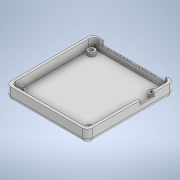
# Autodesk Inventor part: Enclosure Box
Saved by Autodesk Inventor 2021 (Build 250183000, 183)
## iProperties
Created: 2021-06-04
Part Number: Enclosure Box
Material: Generic
Document SubType Name: Modeling
Designer: Anton
Density: 1 g/cm^3
Appearance: Default
Author: Anton
Autodesk Inventor part; units mm, degrees
ref_plane "YZ Plane" through (0, 0, 0) normal (1, 0, 0) x (0, 1, 0)
ref_plane "XZ Plane" through (0, 0, 0) normal (0, 1, 0) x (-1, 0, 0)
ref_plane "XY Plane" through (0, 0, 0) normal (0, 0, 1) x (1, 0, 0)
sketch "Sketch2" plane through (0, 0, 0) normal (0, 1, 0) x (-1, 0, 0)
  line L0 (0, 0) -> (62, 0)
  line L1 (62, 0) -> (62, -66)
  line L2 (62, -66) -> (0, -66)
  line L3 (0, -66) -> (0, 0)
  circle A0 centre (58.15, -9.3) radius 1.5
  circle A1 centre (57.35, -60.86) radius 1.5
  circle A2 centre (3, -4.5) radius 1.5
  circle A3 centre (3, -61.9) radius 1.5
  circle A4 centre (3, -4.5) radius 3
  circle A5 centre (58.15, -9.3) radius 3
  circle A6 centre (57.35, -60.86) radius 3
  circle A7 centre (3, -61.9) radius 3
  line L4 (63, 20) -> (-1, 20)
  line L5 (-1, 20) -> (-1, -86)
  line L6 (-1, -86) -> (63, -86)
  line L7 (63, -86) -> (63, 20)
  dimension "d14" = 66
  dimension "d15" = 62
  dimension "d16" = 3
  dimension "d17" = 3
  dimension "d18" = 3
  dimension "d19" = 3
  dimension "d20" = 3
  dimension "d21" = 4.5
  dimension "d22" = 6
  dimension "d23" = 3
  dimension "d24" = 57.4
  dimension "d25" = 54.35
  dimension "d26" = 0.8
  dimension "d27" = 51.56
  dimension "d28" = 4.8
  dimension "d29" = 6
  dimension "d30" = 6
  dimension "d31" = 6
  dimension "d32" = 20
  dimension "d33" = 20
  dimension "d34" = 1
  dimension "d35" = 1
  constraints: 16 end point, 8 centre point, 4 coincident, 4 parallel, 2 horizontal, 2 perpendicular
  measures "d14" distance between parallel lines of L2 L0
  measures "d15" distance between parallel lines of L3 L1
  measures "d16" diameter of A0
  measures "d17" diameter of A1
  measures "d18" diameter of A3
  measures "d19" diameter of A2
  measures "d20" distance from line of L3 A2.centre
  measures "d21" distance from line of A2.centre L0
  measures "d22" diameter of A4
  measures "d23" distance from line of L3 A3.centre
  measures "d24" distance of A2.centre A3.centre
  measures "d25" horizontal distance of A1.centre A3.centre
  measures "d26" horizontal distance of A1.centre A0.centre
  measures "d27" vertical distance of A1.centre A0.centre
  measures "d28" vertical distance of A2.centre A0.centre
  measures "d29" diameter of A5
  measures "d30" diameter of A6
  measures "d31" diameter of A7
  measures "d32" distance between parallel lines of L4 L0
  measures "d33" distance between parallel lines of L2 L6
  measures "d34" distance between parallel lines of L7 L1
  measures "d35" distance between parallel lines of L3 L5
extrude "Extrusion1" add sketch "Sketch2" along normal blind 2 contours A4 | A7 | L0 L1 L2 L3 | A0 | A1 | A2 | A3 | A5 | A6
sketch "Sketch4" plane through (0, 2, 0) normal (0, 1, 0) x (1, 0, 0)
  line L0 (-62, 66) -> (0, 66)
  line L1 (0, 66) -> (0, 0)
  line L2 (0, 0) -> (-62, 0)
  line L3 (-62, 0) -> (-62, 66)
  circle A0 centre (-3.85, 56.7) radius 1.5
  circle A1 centre (-4.65, 5.14) radius 1.5
  circle A2 centre (-59, 61.5) radius 1.5
  circle A3 centre (-59, 4.1) radius 1.5
  circle A4 centre (-59, 61.5) radius 3
  circle A5 centre (-3.85, 56.7) radius 3
  circle A6 centre (-4.65, 5.14) radius 3
  circle A7 centre (-59, 4.1) radius 3
  point P0 (0, 0)
  dimension "d38" = 66
  dimension "d40" = 3
  dimension "d41" = 3
  dimension "d42" = 3
  dimension "d43" = 3
  dimension "d44" = 3
  dimension "d45" = 4.5
  dimension "d46" = 6
  dimension "d47" = 3
  dimension "d48" = 57.4
  dimension "d50" = 0.8
  dimension "d51" = 51.56
  dimension "d52" = 4.8
  dimension "d53" = 6
  dimension "d54" = 6
  dimension "d55" = 6
  constraints: 8 centre point, 8 end point, 4 coincident, 2 parallel, 1 horizontal, 1 perpendicular
  measures "d38" distance between parallel lines of L2 L0
  measures "d40" diameter of A0
  measures "d41" diameter of A1
  measures "d42" diameter of A3
  measures "d43" diameter of A2
  measures "d44" distance from line of L3 A2.centre
  measures "d45" distance from line of A2.centre L0
  measures "d46" diameter of A4
  measures "d47" distance from line of L3 A3.centre
  measures "d48" distance of A2.centre A3.centre
  measures "d50" horizontal distance of A1.centre A0.centre
  measures "d51" vertical distance of A1.centre A0.centre
  measures "d52" vertical distance of A2.centre A0.centre
  measures "d53" diameter of A5
  measures "d54" diameter of A6
  measures "d55" diameter of A7
extrude "Extrusion2" add sketch "Sketch4" along normal blind 3 contours A4 | A7 | A0 | A1 | A2 | A3 | A5 | A6
sketch "Sketch69" plane through (-59, 5, -4.1) normal (0, 1, 0) x (1, 0, 0)
  circle A0 centre (54.35, 1.04) radius 3 projected
  circle A1 centre (54.35, 1.04) radius 1.25
  circle A2 centre (55.15, 52.6) radius 3 projected
  circle A3 centre (55.15, 52.6) radius 1.25
  circle A4 centre (0, 57.4) radius 3 projected
  circle A5 centre (0, 57.4) radius 1.25
  circle A6 centre (0, 0) radius 3 projected
  circle A7 centre (0, 0) radius 1.25
  point P0 (59, -4.1)
  point P1 (-3, 57.4)
  point P2 (-3, 0)
  dimension "d432" = 2.5
  dimension "d433" = 2.5
  dimension "d434" = 2.5
  dimension "d435" = 2.5
  constraints: 4 centre point, 4 coincident, 2 horizontal alignment
  measures "d432" diameter of A7
  measures "d433" diameter of A5
  measures "d434" diameter of A3
  measures "d435" diameter of A1
extrude "Extrusion56" add sketch "Sketch69" along normal blind 3 contours A1 | A3 | A5 | A7
sketch "Sketch72" plane through (0, 2, 0) normal (0, 1, 0) x (1, 0, 0)
  line L0 (-62, 66) -> (-62, 0) projected
  line L1 (-62, 66) -> (-65, 66)
  line L2 (-65, 66) -> (-65, 0)
  line L3 (-65, 0) -> (-62, 0)
  line L4 (-62, 0) -> (-62, 66)
  circle A0 centre (-59, 61.5) radius 1.25 projected
  line L5 (0, 66) -> (-62, 66) projected
  line L6 (-62, 0) -> (0, 0) projected
  line L7 (0, 0) -> (2.15, 0)
  line L8 (2.15, 0) -> (2.15, 66)
  line L9 (2.15, 66) -> (0, 66)
  line L10 (0, 66) -> (0, 0)
  circle A1 centre (-3.85, 56.7) radius 1.25 projected
  line L11 (-65, 66) -> (2.15, 66)
  line L12 (2.15, 66) -> (2.15, 68.5)
  line L13 (2.15, 68.5) -> (-65, 68.5)
  line L14 (-65, 68.5) -> (-65, 66)
  line L15 (-65, 0) -> (2.15, 0)
  line L16 (2.15, 0) -> (2.15, -3)
  line L17 (2.15, -3) -> (-65, -3)
  line L18 (-65, -3) -> (-65, 0)
  circle A2 centre (-59, 4.1) radius 1.25 projected
  dimension "d446" = 6
  dimension "d447" = 0
  dimension "d448" = 6
  dimension "d449" = 7
  dimension "d450" = 7.1
  dimension "d464" = 0
  dimension "d465" = 0
  constraints: 32 end point, 8 parallel, 4 horizontal, 4 perpendicular, 1 point on line
  measures "d446" distance from line of A0.centre L2
  measures "d447" distance between parallel lines of L5 L1
  measures "d448" distance from line of L8 A1.centre
  measures "d449" distance from line of A0.centre L13
  measures "d450" distance from line of L17 A2.centre
  measures "d464" distance between parallel lines of L8 L12
  measures "d465" distance between parallel lines of L8 L16
extrude "Extrusion58" add sketch "Sketch72" against normal blind 2 contours L0 L3 L2 L1 | L1 L14 L13 L12 L9 L5 | L6 L7 L16 L17 L18 L3 | L9 L8 L7 L10
sketch "Sketch73" plane through (0, 2, 0) normal (0, 1, 0) x (1, 0, 0)
  line L0 (2.15, -3) -> (-65, -3) projected
  line L1 (-65, 68.5) -> (2.15, 68.5) projected
  line L2 (-65, -3) -> (2.15, -3)
  line L3 (2.15, -3) -> (2.15, 68.5)
  line L4 (2.15, 68.5) -> (-65, 68.5)
  line L5 (-65, 68.5) -> (-65, -3)
  line L6 (-63, -1) -> (0.15, -1)
  line L7 (0.15, -1) -> (0.15, 66.5)
  line L8 (0.15, 66.5) -> (-63, 66.5)
  line L9 (-63, 66.5) -> (-63, -1)
  point P0 (0, 0)
  point P1 (2.15, -3)
  dimension "d453" = 2
  constraints: 16 end point, 4 parallel, 2 perpendicular, 1 horizontal, 3 other
  measures "d453" distance between parallel lines of L5 L9
extrude "Extrusion59" add sketch "Sketch73" along normal blind 6
sketch "Sketch74" plane through (0, 8, 0) normal (0, 1, 0) x (1, 0, 0)
  line L0 (6.1553, 52.4) -> (-1.961, 52.4)
  line L1 (-1.961, 52.4) -> (-1.961, 40.4)
  line L2 (-1.961, 40.4) -> (6.1553, 40.4)
  line L3 (6.1553, 40.4) -> (6.1553, 52.4)
  line L4 (-3.5, 77.4858) -> (-56, 77.4858)
  line L5 (-56, 77.4858) -> (-56, 63.7045)
  line L6 (-56, 63.7045) -> (-3.5, 63.7045)
  line L7 (-3.5, 63.7045) -> (-3.5, 77.4858)
  circle A0 centre (-59, 61.5) radius 1.25 projected
  line L8 (0.15, -1) -> (0.15, 66.5) projected
  line L9 (-63, 67.5) -> (0.15, 67.5)
  line L10 (0.15, 67.5) -> (0.15, 64.6943)
  line L11 (0.15, 64.6943) -> (-63, 64.6943)
  line L12 (-63, 64.6943) -> (-63, 67.5)
  line L13 (-63, 66.5) -> (0.15, 66.5) projected
  circle A1 centre (-3.85, 56.7) radius 1.25 projected
  point P0 (0, 0)
  point P1 (-56, 64.6943)
  point P2 (-3.5, 64.6943)
  point P3 (-56, 66.5)
  point P4 (-56, 67.5)
  point P5 (-3.5, 66.5)
  point P6 (0.15, 66.5)
  point P7 (-3.5, 67.5)
  dimension "d457" = 52.5
  dimension "d458" = 1
  dimension "d459" = 4.3
  dimension "d460" = 12
  dimension "d463" = 3
  constraints: 24 end point, 6 parallel, 3 horizontal, 3 perpendicular, 1 point on line
  measures "d457" distance between parallel lines of L7 L5
  measures "d458" distance between parallel lines of L13 L9
  measures "d459" distance from line of L0 A1.centre
  measures "d460" distance between parallel lines of L0 L2
  measures "d463" distance from line of L5 A0.centre
extrude "Extrusion60" cut sketch "Sketch74" against normal blind 3 contours L3 L2 L8 L0 | L8 L2 L1 L0 | L13 L7 L9 L10 | L11 L5 L13 L7 | L13 L5 L9 L7 | L9 L5 L4 L7 | L13 L12 L9 L5
sketch "Sketch75" plane through (0, 5, 0) normal (0, 1, 0) x (1, 0, 0)
  line L0 (-56, 68.5) -> (-3.5, 68.5) projected
  line L1 (-56, 68.5) -> (-3.5, 68.5)
  line L2 (-3.5, 68.5) -> (-3.5, 67.5)
  line L3 (-3.5, 67.5) -> (-56, 67.5)
  line L4 (-56, 67.5) -> (-56, 68.5)
  point P0 (0, 0)
  point P1 (-3.5, 68.5)
  constraints: 8 end point, 2 parallel, 1 horizontal, 1 perpendicular
extrude "Extrusion61" add sketch "Sketch75" along normal blind 1.5
sketch "Sketch77" plane through (0, 5, 0) normal (0, 1, 0) x (1, 0, 0)
  line L0 (2.15, 52.4) -> (2.15, 68.5) projected
  line L1 (2.15, 40.4) -> (0.15, 40.4) projected
  line L2 (2.15, 52.4) -> (1.15, 52.4)
  line L3 (1.15, 52.4) -> (1.15, 40.4)
  line L4 (1.15, 40.4) -> (2.15, 40.4)
  line L5 (2.15, 40.4) -> (2.15, 52.4)
  point P0 (0, 0)
  dimension "d469" = 1
  constraints: 8 end point, 2 parallel, 1 horizontal, 1 midpoint, 1 perpendicular
  measures "d469" distance between parallel lines of L5 L3
extrude "Extrusion62" add sketch "Sketch77" along normal blind 1.5
sketch "Sketch78" plane through (0, 8, 0) normal (0, 1, 0) x (1, 0, 0)
  line L0 (2.15, 40.4) -> (0.15, 40.4) projected
  line L1 (0.15, 40.4) -> (0.15, -1) projected
  line L2 (0.15, -1) -> (-63, -1) projected
  line L3 (-63, -1) -> (-63, 67.5) projected
  line L4 (-63, 67.5) -> (-56, 67.5) projected
  line L5 (-56, 67.5) -> (-56, 68.5) projected
  line L6 (-56, 68.5) -> (-65, 68.5) projected
  line L7 (-65, 68.5) -> (-65, -3) projected
  line L8 (-65, -3) -> (2.15, -3) projected
  line L9 (2.15, -3) -> (2.15, 40.4) projected
  line L10 (0.15, 52.4) -> (2.15, 52.4) projected
  line L11 (2.15, 52.4) -> (2.15, 68.5) projected
  line L12 (2.15, 68.5) -> (-3.5, 68.5) projected
  line L13 (-3.5, 68.5) -> (-3.5, 67.5) projected
  line L14 (-3.5, 67.5) -> (0.15, 67.5) projected
  line L15 (0.15, 67.5) -> (0.15, 52.4) projected
  point P0 (0, 0)
extrude "Extrusion63" add sketch "Sketch78" along normal blind 2
sketch "Sketch80" plane through (0, 10, 0) normal (0, 1, 0) x (1, 0, 0)
  line L0 (2.15, -3) -> (-65, -3) projected
  line L1 (-1.85, -3) -> (-61, -3)
  line L2 (-65, 1) -> (-65, 64.5)
  line L3 (-61, 68.5) -> (-1.85, 68.5)
  line L4 (2.15, 64.5) -> (2.15, 1)
  line L5 (-68.7627, 72.319) -> (6.3795, 72.319)
  line L6 (6.3795, 72.319) -> (6.3795, -5.0493)
  line L7 (6.3795, -5.0493) -> (-68.7627, -5.0493)
  line L8 (-68.7627, -5.0493) -> (-68.7627, 72.319)
  arc A0 (-61, 68.5) -> (-65, 64.5) centre (-61, 64.5) ccw
  arc A1 (2.15, 64.5) -> (-1.85, 68.5) centre (-1.85, 64.5) ccw
  arc A2 (-1.85, -3) -> (2.15, 1) centre (-1.85, 1) ccw
  arc A3 (-65, 1) -> (-61, -3) centre (-61, 1) ccw
  point P0 (0, 0)
  point P1 (-65, 68.5)
  dimension "d475" = 4
  constraints: 16 end point, 8 point on circle, 8 tangent, 4 centre point, 4 parallel, 4 point on line, 3 equal radius, 2 horizontal, 2 perpendicular
  measures "d475" radius of A0
extrude "Extrusion64" cut sketch "Sketch80" against normal blind 10
sketch "Sketch81" plane through (0, 10, 0) normal (0, 1, 0) x (1, 0, 0)
  line L0 (0.15, 40.4) -> (0.15, -1) projected
  line L1 (-63, 66.5) -> (-63, 67.5) projected
  line L2 (-3.85, -1) -> (-59, -1)
  line L3 (-63, 3) -> (-63, 63.5)
  line L4 (-59, 67.5) -> (-3.85, 67.5)
  line L5 (0.15, 63.5) -> (0.15, 3)
  arc A0 (-59, 67.5) -> (-63, 63.5) centre (-59, 63.5) ccw
  arc A1 (0.15, 63.5) -> (-3.85, 67.5) centre (-3.85, 63.5) ccw
  arc A2 (-3.85, -1) -> (0.15, 3) centre (-3.85, 3) ccw
  arc A3 (-63, 3) -> (-59, -1) centre (-59, 3) ccw
  line L6 (0.15, -1) -> (-63, -1) projected
  line L7 (-63, 67.5) -> (0.15, 67.5)
  line L8 (0.15, 67.5) -> (0.15, -1)
  line L9 (0.15, -1) -> (-63, -1)
  line L10 (-63, -1) -> (-63, 67.5)
  point P0 (0, 0)
  dimension "d478" = 4
  constraints: 16 end point, 8 point on circle, 8 tangent, 4 centre point, 4 parallel, 4 point on line, 3 equal radius, 2 horizontal, 2 perpendicular
  measures "d478" radius of A0
extrude "Extrusion65" add sketch "Sketch81" against normal up to surface (8 mm away) contours L0 L6 A2 | A1 L7 L8 | L6 L10 A3 | A0 L10 L1 L7
sketch "Sketch82" plane through (0, 0, 0) normal (0, -1, 0) x (1, 0, 0)
  arc A0 (-61, 3) -> (-65, -1) centre (-61, -1) ccw projected
  line L0 (-65, -1) -> (-65, -64.5) projected
  arc A1 (-65, -64.5) -> (-61, -68.5) centre (-61, -64.5) ccw projected
  line L1 (-61, -68.5) -> (-1.85, -68.5) projected
  arc A2 (-1.85, -68.5) -> (2.15, -64.5) centre (-1.85, -64.5) ccw projected
  line L2 (2.15, -64.5) -> (2.15, -1) projected
  arc A3 (2.15, -1) -> (-1.85, 3) centre (-1.85, -1) ccw projected
  line L3 (-1.85, 3) -> (-61, 3) projected
  point P0 (0, 0)
extrude "Extrusion66" add sketch "Sketch82" along normal blind 1
sketch "Sketch83" plane through (-59, 5, -4.1) normal (0, 1, 0) x (1, 0, 0)
  circle A0 centre (54.35, 1.04) radius 1.25 projected
  circle A1 centre (54.35, 1.04) radius 1.5
  circle A2 centre (55.15, 52.6) radius 1.25 projected
  circle A3 centre (55.15, 52.6) radius 1.5
  circle A4 centre (0, 57.4) radius 1.25 projected
  circle A5 centre (0, 57.4) radius 1.5
  circle A6 centre (0, 0) radius 1.25 projected
  circle A7 centre (0, 0) radius 1.5
  point P0 (59, -4.1)
  dimension "d484" = 3
  dimension "d486" = 3
  dimension "d487" = 3
  dimension "d488" = 3
  constraints: 4 centre point, 4 coincident
  measures "d484" diameter of A7
  measures "d486" diameter of A5
  measures "d487" diameter of A3
  measures "d488" diameter of A1
extrude "Extrusion67" cut sketch "Sketch83" along normal mid plane 1011 contours A0 | A1 | A2 | A3 | A4 | A5 | A6 | A7
fillet "Fillet13" radius 4 8 edges at (0.9784, -1, -67.3284) (2.15, -1, -32.75) (0.9784, -1, 1.8284) (-31.425, -1, 3) (-63.8284, -1, 1.8284) (-65, -1, -32.75) (-63.8284, -1, -67.3284) (-31.425, -1, -68.5)
sketch "Sketch84" plane through (0, -1, 0) normal (0, -1, 0) x (1, 0, 0)
  circle A0 centre (-4.65, -5.14) radius 3 projected
  circle A1 centre (-4.65, -5.14) radius 3
  circle A2 centre (-3.85, -56.7) radius 1.5 projected
  circle A3 centre (-3.85, -56.7) radius 3
  circle A4 centre (-59, -61.5) radius 1.5 projected
  circle A5 centre (-59, -61.5) radius 3
  circle A6 centre (-59, -4.1) radius 1.5 projected
  circle A7 centre (-59, -4.1) radius 3
  point P0 (0, 0)
  dimension "d492" = 6
  dimension "d493" = 6
  dimension "d494" = 6
  dimension "d495" = 6
  constraints: 4 centre point, 4 coincident
  measures "d492" diameter of A7
  measures "d493" diameter of A5
  measures "d494" diameter of A3
  measures "d495" diameter of A1
extrude "Extrusion68" cut sketch "Sketch84" against normal blind 2.5 contours A0 | A2 | A3 | A4 | A5 | A7
sketch "Sketch86" plane through (-3.5, 6.5, -68.5) normal (0, 0, -1) x (-1, 0, 0)
  line L0 (0, 0) -> (0, 3.5) projected
  line L1 (57.5, -3.5) -> (-1.65, -3.5) projected
  line L2 (0, 0) -> (52.5, 0)
  line L3 (52.5, 0) -> (52.5, -3.5)
  line L4 (52.5, -3.5) -> (0, -3.5)
  line L5 (0, -3.5) -> (0, 0)
  line L6 (52.5, 3.5) -> (52.5, 0) projected
  line L7 (0, 0) -> (52.5, 0) projected
  line L8 (2.1, 0) -> (2.1, -3.5)
  line L9 (4.64, 0) -> (4.64, -3.5)
  line L10 (7.18, 0) -> (7.18, -3.5)
  line L11 (9.72, 0) -> (9.72, -3.5)
  line L12 (12.26, 0) -> (12.26, -3.5)
  line L13 (14.8, 0) -> (14.8, -3.5)
  line L14 (17.34, 0) -> (17.34, -3.5)
  line L15 (19.88, 0) -> (19.88, -3.5)
  line L16 (22.42, 0) -> (22.42, -3.5)
  line L17 (24.96, 0) -> (24.96, -3.5)
  line L18 (27.5, 0) -> (27.5, -3.5)
  line L19 (30.04, 0) -> (30.04, -3.5)
  line L20 (32.58, 0) -> (32.58, -3.5)
  line L21 (35.12, 0) -> (35.12, -3.5)
  line L22 (37.66, 0) -> (37.66, -3.5)
  line L23 (40.2, 0) -> (40.2, -3.5)
  line L24 (42.74, 0) -> (42.74, -3.5)
  line L25 (45.28, 0) -> (45.28, -3.5)
  line L26 (47.82, 0) -> (47.82, -3.5)
  line L27 (50.36, 0) -> (50.36, -3.5)
  circle A0 centre (50.36, -2) radius 1
  circle A1 centre (24.96, -2) radius 1
  line L28 (47.57, 0) -> (48.07, 0)
  line L29 (48.07, 0) -> (48.07, -3.5)
  line L30 (48.07, -3.5) -> (47.57, -3.5)
  line L31 (47.57, -3.5) -> (47.57, 0)
  line L32 (45.03, 0) -> (45.53, 0)
  line L33 (45.53, 0) -> (45.53, -3.5)
  line L34 (45.53, -3.5) -> (45.03, -3.5)
  line L35 (45.03, -3.5) -> (45.03, 0)
  line L36 (45.53, -3.4) -> (47.57, -3.4)
  line L37 (42.49, 0) -> (42.99, 0)
  line L38 (42.99, 0) -> (42.99, -3.5)
  line L39 (42.99, -3.5) -> (42.49, -3.5)
  line L40 (42.49, -3.5) -> (42.49, 0)
  line L41 (39.95, 0) -> (40.45, 0)
  line L42 (40.45, 0) -> (40.45, -3.5)
  line L43 (40.45, -3.5) -> (39.95, -3.5)
  line L44 (39.95, -3.5) -> (39.95, 0)
  line L45 (37.41, 0) -> (37.91, 0)
  line L46 (37.91, 0) -> (37.91, -3.5)
  line L47 (37.91, -3.5) -> (37.41, -3.5)
  line L48 (37.41, -3.5) -> (37.41, 0)
  line L49 (34.87, 0) -> (35.37, 0)
  line L50 (35.37, 0) -> (35.37, -3.5)
  line L51 (35.37, -3.5) -> (34.87, -3.5)
  line L52 (34.87, -3.5) -> (34.87, 0)
  line L53 (32.33, 0) -> (32.83, 0)
  line L54 (32.83, 0) -> (32.83, -3.5)
  line L55 (32.83, -3.5) -> (32.33, -3.5)
  line L56 (32.33, -3.5) -> (32.33, 0)
  line L57 (29.79, 0) -> (30.29, 0)
  line L58 (30.29, 0) -> (30.29, -3.5)
  line L59 (30.29, -3.5) -> (29.79, -3.5)
  line L60 (29.79, -3.5) -> (29.79, 0)
  line L61 (27.25, 0) -> (27.75, 0)
  line L62 (27.75, -3.5) -> (27.25, -3.5)
  line L63 (40.45, -3.4) -> (42.49, -3.4)
  line L64 (37.41, -3.4) -> (35.37, -3.4)
  line L65 (32.33, -3.4) -> (30.29, -3.4)
  line L66 (22.17, 0) -> (22.67, 0)
  line L67 (22.67, 0) -> (22.67, -3.5)
  line L68 (22.67, -3.5) -> (22.17, -3.5)
  line L69 (22.17, -3.5) -> (22.17, 0)
  line L70 (19.63, 0) -> (20.13, 0)
  line L71 (20.13, 0) -> (20.13, -3.5)
  line L72 (20.13, -3.5) -> (19.63, -3.5)
  line L73 (19.63, -3.5) -> (19.63, 0)
  line L74 (17.09, 0) -> (17.59, 0)
  line L75 (17.59, 0) -> (17.59, -3.5)
  line L76 (17.59, -3.5) -> (17.09, -3.5)
  line L77 (17.09, -3.5) -> (17.09, 0)
  line L78 (14.55, 0) -> (15.05, 0)
  line L79 (15.05, 0) -> (15.05, -3.5)
  line L80 (15.05, -3.5) -> (14.55, -3.5)
  line L81 (14.55, -3.5) -> (14.55, 0)
  line L82 (12.01, 0) -> (12.51, 0)
  line L83 (12.51, 0) -> (12.51, -3.5)
  line L84 (12.51, -3.5) -> (12.01, -3.5)
  line L85 (12.01, -3.5) -> (12.01, 0)
  line L86 (9.47, 0) -> (9.97, 0)
  line L87 (9.97, 0) -> (9.97, -3.5)
  line L88 (9.97, -3.5) -> (9.47, -3.5)
  line L89 (9.47, -3.5) -> (9.47, 0)
  line L90 (6.8118, 0) -> (7.7537, 0)
  line L91 (7.7537, -3.5) -> (6.8118, -3.5)
  line L92 (22.17, -3.4) -> (20.13, -3.4)
  line L93 (17.09, -3.4) -> (15.05, -3.4)
  line L94 (12.01, -3.4) -> (9.97, -3.4)
  line L95 (0, -3.4) -> (2.1, -3.4)
  line L96 (4.64, -3.4) -> (2.1, -3.4)
  line L97 (47.3552, -3.4) -> (45.8683, -3.4)
  line L98 (45.8683, -3.4) -> (45.8683, -3.0888)
  line L99 (45.8683, -3.0888) -> (46.4216, -3.0888)
  line L100 (46.4216, -3.0888) -> (46.4216, -1.0461)
  line L101 (46.4216, -1.0461) -> (45.8683, -1.0461)
  line L102 (45.8683, -1.0461) -> (45.8683, -0.767)
  spline S0 degree 2 poles (45.8683, -0.767) (46.182, -0.767) (46.4784, -0.5891) (46.4981, -0.3421) knots 0 0 0 1 2 2 2
  line L103 (46.4981, -0.3421) -> (46.8143, -0.3421)
  line L104 (46.8143, -0.3421) -> (46.8143, -3.0888)
  line L105 (46.8143, -3.0888) -> (47.3552, -3.0888)
  line L106 (47.3552, -3.0888) -> (47.3552, -3.4)
  line L107 (42.4284, -3.4) -> (40.5487, -3.4)
  line L108 (40.5487, -3.4) -> (40.5487, -2.9677)
  spline S1 degree 2 poles (40.5487, -2.9677) (40.7512, -2.7776) (41.1118, -2.4243) (41.2847, -2.2342) knots 0 0 0 1 2 2 2
  spline S2 degree 2 poles (41.2847, -2.2342) (41.633, -1.8513) (41.8874, -1.3919) (41.8874, -1.1473) knots 0 0 0 1 2 2 2
  spline S3 degree 2 poles (41.8874, -1.1473) (41.8874, -1.0189) (41.8084, -0.8262) (41.7368, -0.7645) knots 0 0 0 1 2 2 2
  spline S4 degree 2 poles (41.7368, -0.7645) (41.6651, -0.7027) (41.4774, -0.641) (41.3638, -0.641) knots 0 0 0 1 2 2 2
  spline S5 degree 2 poles (41.3638, -0.641) (41.2551, -0.641) (41.0328, -0.6953) (40.9315, -0.7373) knots 0 0 0 1 2 2 2
  spline S6 degree 2 poles (40.9315, -0.7373) (40.8451, -0.7719) (40.6845, -0.8707) (40.6351, -0.9053) knots 0 0 0 1 2 2 2
  line L109 (40.6351, -0.9053) -> (40.6129, -0.9053)
  line L110 (40.6129, -0.9053) -> (40.6129, -0.4706)
  spline S7 degree 2 poles (40.6129, -0.4706) (40.7389, -0.4088) (41.1909, -0.2878) (41.3934, -0.2878) knots 0 0 0 1 2 2 2
  spline S8 degree 2 poles (41.3934, -0.2878) (41.8207, -0.2878) (42.3024, -0.7398) (42.3024, -1.1251) knots 0 0 0 1 2 2 2
  spline S9 degree 2 poles (42.3024, -1.1251) (42.3024, -1.3054) (42.2184, -1.6068) (42.1443, -1.7352) knots 0 0 0 1 2 2 2
  spline S10 degree 2 poles (42.1443, -1.7352) (42.0702, -1.8686) (41.8553, -2.1304) (41.7368, -2.2564) knots 0 0 0 1 2 2 2
  spline S11 degree 2 poles (41.7368, -2.2564) (41.5441, -2.4663) (41.0723, -2.9159) (40.9315, -3.0468) knots 0 0 0 1 2 2 2
  line L111 (40.9315, -3.0468) -> (42.4284, -3.0468)
  line L112 (42.4284, -3.0468) -> (42.4284, -3.4)
  spline S12 degree 2 poles (36.2912, -0.641) (36.18, -0.641) (35.9602, -0.6953) (35.854, -0.7373) knots 0 0 0 1 2 2 2
  spline S13 degree 2 poles (35.854, -0.7373) (35.7552, -0.7793) (35.6095, -0.8682) (35.5527, -0.9078) knots 0 0 0 1 2 2 2
  line L113 (35.5527, -0.9078) -> (35.528, -0.9078)
  line L114 (35.528, -0.9078) -> (35.528, -0.4755)
  spline S14 degree 2 poles (35.528, -0.4755) (35.6613, -0.4039) (36.1183, -0.2878) (36.3233, -0.2878) knots 0 0 0 1 2 2 2
  spline S15 degree 2 poles (36.3233, -0.2878) (36.5308, -0.2878) (36.8395, -0.3718) (36.9655, -0.4607) knots 0 0 0 1 2 2 2
  spline S16 degree 2 poles (36.9655, -0.4607) (37.0989, -0.557) (37.2372, -0.8361) (37.2372, -1.0238) knots 0 0 0 1 2 2 2
  spline S17 degree 2 poles (37.2372, -1.0238) (37.2372, -1.2758) (36.9062, -1.6562) (36.6741, -1.7056) knots 0 0 0 1 2 2 2
  line L115 (36.6741, -1.7056) -> (36.6741, -1.7352)
  spline S18 degree 2 poles (36.6741, -1.7352) (36.7704, -1.755) (36.9902, -1.8439) (37.0841, -1.9328) knots 0 0 0 1 2 2 2
  spline S19 degree 2 poles (37.0841, -1.9328) (37.1779, -2.0193) (37.2965, -2.2959) (37.2965, -2.496) knots 0 0 0 1 2 2 2
  spline S20 degree 2 poles (37.2965, -2.496) (37.2965, -2.701) (37.1557, -3.0493) (37.0273, -3.1826) knots 0 0 0 1 2 2 2
  spline S21 degree 2 poles (37.0273, -3.1826) (36.8939, -3.321) (36.516, -3.4642) (36.2764, -3.4642) knots 0 0 0 1 2 2 2
  spline S22 degree 2 poles (36.2764, -3.4642) (36.0467, -3.4642) (35.5971, -3.3531) (35.444, -3.2765) knots 0 0 0 1 2 2 2
  line L116 (35.444, -3.2765) -> (35.444, -2.8442)
  line L117 (35.444, -2.8442) -> (35.4736, -2.8442)
  spline S23 degree 2 poles (35.4736, -2.8442) (35.6021, -2.9381) (36.0368, -3.111) (36.2517, -3.111) knots 0 0 0 1 2 2 2
  spline S24 degree 2 poles (36.2517, -3.111) (36.3776, -3.111) (36.6296, -3.032) (36.7136, -2.9406) knots 0 0 0 1 2 2 2
  spline S25 degree 2 poles (36.7136, -2.9406) (36.7951, -2.8492) (36.8815, -2.6318) (36.8815, -2.4663) knots 0 0 0 1 2 2 2
  spline S26 degree 2 poles (36.8815, -2.4663) (36.8815, -2.3008) (36.7852, -2.086) (36.6988, -2.0242) knots 0 0 0 1 2 2 2
  spline S27 degree 2 poles (36.6988, -2.0242) (36.6123, -1.9625) (36.3776, -1.9155) (36.2393, -1.9155) knots 0 0 0 1 2 2 2
  line L118 (36.2393, -1.9155) -> (36.0664, -1.9155)
  line L119 (36.0664, -1.9155) -> (36.0664, -1.5771)
  line L120 (36.0664, -1.5771) -> (36.2023, -1.5771)
  spline S28 degree 2 poles (36.2023, -1.5771) (36.4765, -1.5771) (36.8223, -1.3153) (36.8223, -1.0658) knots 0 0 0 1 2 2 2
  spline S29 degree 2 poles (36.8223, -1.0658) (36.8223, -0.9497) (36.7333, -0.7843) (36.6617, -0.7349) knots 0 0 0 1 2 2 2
  spline S30 degree 2 poles (36.6617, -0.7349) (36.5851, -0.683) (36.3974, -0.641) (36.2912, -0.641) knots 0 0 0 1 2 2 2
  line L121 (32.3499, -2.3527) -> (31.9868, -2.3527)
  line L122 (31.9868, -2.3527) -> (31.9868, -3.4)
  line L123 (31.9868, -3.4) -> (31.5941, -3.4)
  line L124 (31.5941, -3.4) -> (31.5941, -2.3527)
  line L125 (31.5941, -2.3527) -> (30.2479, -2.3527)
  line L126 (30.2479, -2.3527) -> (30.2479, -1.9229)
  line L127 (30.2479, -1.9229) -> (31.6113, -0.352)
  line L128 (31.6113, -0.352) -> (31.9868, -0.352)
  line L129 (31.9868, -0.352) -> (31.9868, -2.0242)
  line L130 (31.9868, -2.0242) -> (32.3499, -2.0242)
  line L131 (32.3499, -2.0242) -> (32.3499, -2.3527)
  line L132 (31.5941, -2.0242) -> (31.5941, -0.8337)
  line L133 (31.5941, -0.8337) -> (30.569, -2.0242)
  line L134 (30.569, -2.0242) -> (31.5941, -2.0242)
  spline S31 degree 2 poles (22.0763, -2.4318) (22.0763, -2.6516) (21.9355, -3.027) (21.807, -3.1653) knots 0 0 0 1 2 2 2
  spline S32 degree 2 poles (21.807, -3.1653) (21.6786, -3.3037) (21.2957, -3.4642) (21.0586, -3.4642) knots 0 0 0 1 2 2 2
  spline S33 degree 2 poles (21.0586, -3.4642) (20.8412, -3.4642) (20.4164, -3.3679) (20.2608, -3.2913) knots 0 0 0 1 2 2 2
  line L135 (20.2608, -3.2913) -> (20.2608, -2.8591)
  line L136 (20.2608, -2.8591) -> (20.2904, -2.8591)
  spline S34 degree 2 poles (20.2904, -2.8591) (20.3374, -2.8936) (20.5127, -2.9826) (20.6189, -3.0221) knots 0 0 0 1 2 2 2
  spline S35 degree 2 poles (20.6189, -3.0221) (20.74, -3.0641) (20.94, -3.111) (21.066, -3.111) knots 0 0 0 1 2 2 2
  spline S36 degree 2 poles (21.066, -3.111) (21.1895, -3.111) (21.4217, -3.0221) (21.5057, -2.9258) knots 0 0 0 1 2 2 2
  spline S37 degree 2 poles (21.5057, -2.9258) (21.5823, -2.8344) (21.6613, -2.5923) (21.6613, -2.4293) knots 0 0 0 1 2 2 2
  spline S38 degree 2 poles (21.6613, -2.4293) (21.6613, -2.2663) (21.5724, -2.0588) (21.4884, -1.9896) knots 0 0 0 1 2 2 2
  spline S39 degree 2 poles (21.4884, -1.9896) (21.4019, -1.9131) (21.1451, -1.8488) (20.9894, -1.8488) knots 0 0 0 1 2 2 2
  spline S40 degree 2 poles (20.9894, -1.8488) (20.8215, -1.8488) (20.488, -1.9007) (20.3868, -1.9229) knots 0 0 0 1 2 2 2
  line L137 (20.3868, -1.9229) -> (20.3868, -0.352)
  line L138 (20.3868, -0.352) -> (22.059, -0.352)
  line L139 (22.059, -0.352) -> (22.059, -0.7102)
  line L140 (22.059, -0.7102) -> (20.7795, -0.7102)
  line L141 (20.7795, -0.7102) -> (20.7795, -1.5228)
  spline S41 degree 2 poles (20.7795, -1.5228) (20.8536, -1.5129) (20.9969, -1.5055) (21.0561, -1.5055) knots 0 0 0 1 2 2 2
  spline S42 degree 2 poles (21.0561, -1.5055) (21.2908, -1.5055) (21.6144, -1.5821) (21.7626, -1.6957) knots 0 0 0 1 2 2 2
  spline S43 degree 2 poles (21.7626, -1.6957) (21.9132, -1.8093) (22.0763, -2.1551) (22.0763, -2.4318) knots 0 0 0 1 2 2 2
  spline S44 degree 2 poles (17.0753, -2.412) (17.0753, -2.6466) (16.9197, -3.0443) (16.7888, -3.1777) knots 0 0 0 1 2 2 2
  spline S45 degree 2 poles (16.7888, -3.1777) (16.6529, -3.3185) (16.3121, -3.4642) (16.1071, -3.4642) knots 0 0 0 1 2 2 2
  spline S46 degree 2 poles (16.1071, -3.4642) (15.902, -3.4642) (15.5636, -3.3259) (15.4352, -3.1876) knots 0 0 0 1 2 2 2
  spline S47 degree 2 poles (15.4352, -3.1876) (15.2771, -3.0221) (15.0993, -2.4663) (15.0993, -2.0613) knots 0 0 0 1 2 2 2
  spline S48 degree 2 poles (15.0993, -2.0613) (15.0993, -1.6636) (15.2623, -1.0238) (15.4327, -0.7867) knots 0 0 0 1 2 2 2
  spline S49 degree 2 poles (15.4327, -0.7867) (15.5982, -0.5545) (16.1219, -0.2952) (16.4652, -0.2952) knots 0 0 0 1 2 2 2
  spline S50 degree 2 poles (16.4652, -0.2952) (16.5665, -0.2952) (16.7443, -0.3149) (16.811, -0.3372) knots 0 0 0 1 2 2 2
  line L142 (16.811, -0.3372) -> (16.811, -0.7299)
  line L143 (16.811, -0.7299) -> (16.7937, -0.7299)
  spline S51 degree 2 poles (16.7937, -0.7299) (16.7369, -0.7003) (16.5294, -0.6484) (16.4109, -0.6484) knots 0 0 0 1 2 2 2
  spline S52 degree 2 poles (16.4109, -0.6484) (16.0305, -0.6484) (15.5636, -1.1622) (15.5192, -1.666) knots 0 0 0 1 2 2 2
  spline S53 degree 2 poles (15.5192, -1.666) (15.6649, -1.5648) (15.9712, -1.4536) (16.154, -1.4536) knots 0 0 0 1 2 2 2
  spline S54 degree 2 poles (16.154, -1.4536) (16.3318, -1.4536) (16.5986, -1.5253) (16.7443, -1.6339) knots 0 0 0 1 2 2 2
  spline S55 degree 2 poles (16.7443, -1.6339) (16.9123, -1.7599) (17.0753, -2.1502) (17.0753, -2.412) knots 0 0 0 1 2 2 2
  spline S56 degree 2 poles (16.6603, -2.4293) (16.6603, -2.2416) (16.5615, -1.9872) (16.4529, -1.8982) knots 0 0 0 1 2 2 2
  spline S57 degree 2 poles (16.4529, -1.8982) (16.3713, -1.834) (16.1688, -1.792) (16.0626, -1.792) knots 0 0 0 1 2 2 2
  spline S58 degree 2 poles (16.0626, -1.792) (15.9193, -1.792) (15.6501, -1.8785) (15.5192, -1.96) knots 0 0 0 1 2 2 2
  spline S59 degree 2 poles (15.5192, -1.96) (15.5167, -2.0044) (15.5118, -2.0884) (15.5118, -2.1526) knots 0 0 0 1 2 2 2
  spline S60 degree 2 poles (15.5118, -2.1526) (15.5118, -2.4688) (15.6353, -2.8566) (15.7291, -2.9579) knots 0 0 0 1 2 2 2
  spline S61 degree 2 poles (15.7291, -2.9579) (15.8156, -3.0542) (16.0033, -3.1308) (16.1095, -3.1308) knots 0 0 0 1 2 2 2
  spline S62 degree 2 poles (16.1095, -3.1308) (16.3565, -3.1308) (16.6603, -2.78) (16.6603, -2.4293) knots 0 0 0 1 2 2 2
  line L144 (11.9829, -0.809) -> (10.664, -3.4)
  line L145 (10.664, -3.4) -> (10.2292, -3.4)
  line L146 (10.2292, -3.4) -> (11.6223, -0.7102)
  line L147 (11.6223, -0.7102) -> (10.0489, -0.7102)
  line L148 (10.0489, -0.7102) -> (10.0489, -0.352)
  line L149 (10.0489, -0.352) -> (11.9829, -0.352)
  line L150 (11.9829, -0.352) -> (11.9829, -0.809)
  spline S63 degree 2 poles (4.4126, -1.8212) (4.4084, -1.9941) (4.3446, -2.3173) (4.2746, -2.4449) knots 0 0 0 1 2 2 2
  spline S64 degree 2 poles (4.2746, -2.4449) (4.2047, -2.5684) (3.9968, -2.7249) (3.83, -2.7249) knots 0 0 0 1 2 2 2
  spline S65 degree 2 poles (3.83, -2.7249) (3.7312, -2.7249) (3.5769, -2.6713) (3.5172, -2.6302) knots 0 0 0 1 2 2 2
  spline S66 degree 2 poles (3.5172, -2.6302) (3.4575, -2.587) (3.3484, -2.4676) (3.3052, -2.4161) knots 0 0 0 1 2 2 2
  spline S67 degree 2 poles (3.3052, -2.4161) (3.2599, -2.3605) (3.1714, -2.2432) (3.1281, -2.2) knots 0 0 0 1 2 2 2
  spline S68 degree 2 poles (3.1281, -2.2) (3.0808, -2.1526) (2.982, -2.095) (2.9203, -2.095) knots 0 0 0 1 2 2 2
  spline S69 degree 2 poles (2.9203, -2.095) (2.8338, -2.095) (2.7206, -2.1856) (2.6835, -2.2741) knots 0 0 0 1 2 2 2
  spline S70 degree 2 poles (2.6835, -2.2741) (2.6485, -2.3585) (2.6177, -2.5952) (2.6136, -2.7249) knots 0 0 0 1 2 2 2
  line L151 (2.6136, -2.7249) -> (2.3274, -2.7249)
  spline S71 degree 2 poles (2.3274, -2.7249) (2.3316, -2.5478) (2.3974, -2.2247) (2.4633, -2.1012) knots 0 0 0 1 2 2 2
  spline S72 degree 2 poles (2.4633, -2.1012) (2.5312, -1.9736) (2.7576, -1.8212) (2.912, -1.8212) knots 0 0 0 1 2 2 2
  spline S73 degree 2 poles (2.912, -1.8212) (3.0129, -1.8212) (3.1693, -1.8748) (3.229, -1.918) knots 0 0 0 1 2 2 2
  spline S74 degree 2 poles (3.229, -1.918) (3.2887, -1.9612) (3.3896, -2.0703) (3.4369, -2.13) knots 0 0 0 1 2 2 2
  spline S75 degree 2 poles (3.4369, -2.13) (3.4739, -2.1753) (3.5789, -2.3091) (3.6139, -2.3461) knots 0 0 0 1 2 2 2
  spline S76 degree 2 poles (3.6139, -2.3461) (3.6633, -2.3976) (3.7642, -2.4511) (3.8197, -2.4511) knots 0 0 0 1 2 2 2
  spline S77 degree 2 poles (3.8197, -2.4511) (3.9062, -2.4511) (4.0235, -2.3564) (4.0565, -2.2741) knots 0 0 0 1 2 2 2
  spline S78 degree 2 poles (4.0565, -2.2741) (4.0915, -2.1897) (4.1223, -1.9612) (4.1264, -1.8212) knots 0 0 0 1 2 2 2
  line L152 (4.1264, -1.8212) -> (4.4126, -1.8212)
  spline S79 degree 2 poles (2.0926, -1.8212) (2.0884, -1.9941) (2.0246, -2.3173) (1.9546, -2.4449) knots 0 0 0 1 2 2 2
  spline S80 degree 2 poles (1.9546, -2.4449) (1.8847, -2.5684) (1.6768, -2.7249) (1.51, -2.7249) knots 0 0 0 1 2 2 2
  spline S81 degree 2 poles (1.51, -2.7249) (1.4112, -2.7249) (1.2569, -2.6713) (1.1972, -2.6302) knots 0 0 0 1 2 2 2
  spline S82 degree 2 poles (1.1972, -2.6302) (1.1375, -2.587) (1.0284, -2.4676) (0.9852, -2.4161) knots 0 0 0 1 2 2 2
  spline S83 degree 2 poles (0.9852, -2.4161) (0.9399, -2.3605) (0.8514, -2.2432) (0.8081, -2.2) knots 0 0 0 1 2 2 2
  spline S84 degree 2 poles (0.8081, -2.2) (0.7608, -2.1526) (0.662, -2.095) (0.6003, -2.095) knots 0 0 0 1 2 2 2
  spline S85 degree 2 poles (0.6003, -2.095) (0.5138, -2.095) (0.4006, -2.1856) (0.3635, -2.2741) knots 0 0 0 1 2 2 2
  spline S86 degree 2 poles (0.3635, -2.2741) (0.3285, -2.3585) (0.2977, -2.5952) (0.2936, -2.7249) knots 0 0 0 1 2 2 2
  line L153 (0.2936, -2.7249) -> (0.0074, -2.7249)
  spline S87 degree 2 poles (0.0074, -2.7249) (0.0116, -2.5478) (0.0774, -2.2247) (0.1433, -2.1012) knots 0 0 0 1 2 2 2
  spline S88 degree 2 poles (0.1433, -2.1012) (0.2112, -1.9736) (0.4376, -1.8212) (0.592, -1.8212) knots 0 0 0 1 2 2 2
  spline S89 degree 2 poles (0.592, -1.8212) (0.6929, -1.8212) (0.8493, -1.8748) (0.909, -1.918) knots 0 0 0 1 2 2 2
  spline S90 degree 2 poles (0.909, -1.918) (0.9687, -1.9612) (1.0696, -2.0703) (1.1169, -2.13) knots 0 0 0 1 2 2 2
  spline S91 degree 2 poles (1.1169, -2.13) (1.1539, -2.1753) (1.2589, -2.3091) (1.2939, -2.3461) knots 0 0 0 1 2 2 2
  spline S92 degree 2 poles (1.2939, -2.3461) (1.3433, -2.3976) (1.4442, -2.4511) (1.4997, -2.4511) knots 0 0 0 1 2 2 2
  spline S93 degree 2 poles (1.4997, -2.4511) (1.5862, -2.4511) (1.7035, -2.3564) (1.7365, -2.2741) knots 0 0 0 1 2 2 2
  spline S94 degree 2 poles (1.7365, -2.2741) (1.7715, -2.1897) (1.8023, -1.9612) (1.8064, -1.8212) knots 0 0 0 1 2 2 2
  line L154 (1.8064, -1.8212) -> (2.0926, -1.8212)
  point P0 (-3.5, -6.5)
  point P1 (48.07, 0)
  point P2 (9.97, 0)
  point P3 (12.51, 0)
  point P4 (15.05, 0)
  point P5 (17.59, 0)
  point P6 (20.13, 0)
  point P7 (22.67, 0)
  point P8 (30.29, 0)
  point P9 (32.83, 0)
  point P10 (35.37, 0)
  point P11 (37.91, 0)
  point P12 (37.41, -3.5)
  point P13 (40.45, 0)
  point P14 (39.95, 0)
  point P15 (39.95, -3.5)
  point P16 (42.99, 0)
  dimension "d506" = 0
  dimension "d507" = 2.1
  dimension "d510" = 2.54
  dimension "d515" = 2
  dimension "d516" = 2
  dimension "d517" = 2
  dimension "d518" = 2
  dimension "d519" = 0.25
  dimension "d520" = 0.25
  dimension "d521" = 0.25
  dimension "d522" = 0.25
  dimension "d523" = 0.1
  dimension "d528" = 0.25
  dimension "d529" = 0.25
  dimension "d530" = 0.25
  dimension "d531" = 0.25
  dimension "d532" = 0.25
  dimension "d533" = 0.25
  dimension "d534" = 0.25
  dimension "d535" = 0.25
  dimension "d536" = 0.25
  dimension "d537" = 0.25
  dimension "d538" = 0.25
  dimension "d539" = 0.25
  dimension "d540" = 0.1
  dimension "d541" = 0.1
  dimension "d542" = 0.1
  dimension "d543" = 0.25
  dimension "d544" = 0.25
  dimension "d545" = 0.25
  dimension "d546" = 0.25
  dimension "d547" = 0.25
  dimension "d548" = 0.25
  dimension "d549" = 0.25
  dimension "d550" = 0.25
  dimension "d551" = 0.25
  dimension "d552" = 0.25
  dimension "d553" = 0.25
  dimension "d554" = 0.25
  dimension "d555" = 0.1
  dimension "d556" = 0.1
  dimension "d558" = 0.1
  constraints: 182 end point, 50 parallel, 38 horizontal alignment, 26 horizontal, 22 point on line, 19 perpendicular, 2 centre point, 2 collinear, 2 vertical, 43 other
  measures "d506" distance between parallel lines of L6 L3
  measures "d507" distance between parallel lines of L5 L8
  measures "d510" distance of L8.start L9.start
  measures "d516" diameter of A0
  measures "d517" diameter of A1
  measures "d519" distance between parallel lines of L25 L35
  measures "d520" distance between parallel lines of L25 L33
  measures "d521" distance between parallel lines of L26 L31
  measures "d522" distance between parallel lines of L26 L29
  measures "d528" distance between parallel lines of L19 L60
  measures "d529" distance from line of L19.start L58
  measures "d530" distance between parallel lines of L56 L20
  measures "d531" distance between parallel lines of L20 L54
  measures "d532" distance between parallel lines of L21 L52
  measures "d533" distance between parallel lines of L21 L50
  measures "d534" distance between parallel lines of L22 L48
  measures "d535" distance between parallel lines of L22 L46
  measures "d536" distance between parallel lines of L23 L44
  measures "d537" distance between parallel lines of L23 L42
  measures "d538" distance between parallel lines of L24 L40
  measures "d539" distance between parallel lines of L24 L38
  measures "d543" distance between parallel lines of L16 L69
  measures "d544" distance between parallel lines of L16 L67
  measures "d545" distance between parallel lines of L15 L71
  measures "d546" distance between parallel lines of L15 L73
  measures "d547" distance between parallel lines of L14 L75
  measures "d548" distance between parallel lines of L14 L77
  measures "d549" distance between parallel lines of L13 L79
  measures "d550" distance between parallel lines of L13 L81
  measures "d551" distance between parallel lines of L83 L12
  measures "d552" distance between parallel lines of L12 L85
  measures "d553" distance between parallel lines of L11 L87
  measures "d554" distance between parallel lines of L11 L89
extrude "Extrusion69" cut sketch "Sketch86" against normal blind 0.5 contours L1 L26 L2 L29 | A0 L27 | L27 A0 | L1 L31 L2 L26 | L1 L25 L2 L33 | L1 L35 L2 L25 | L36 L98 L99 L100 L101 L102 S0 L103 L104 L105 L106 | L1 L24 L2 L38 | L1 L40 L2 L24 | L1 L23 L2 L42 | L1 L44 L2 L23 | L63 L108 S1 S2 S3 S4 S5 S6 L109 L110 S7 S8 S9 S10 S11 L111 L112 | L1 L22 L2 L46 | L1 L48 L2 L22 | L1 L21 L2 L50 | L1 L52 L2 L21 | S21 S22 L64 | L64 S22 L116 L117 S23 S24 S25 S26 S27 L118 L119 L120 S28 S29 S30 S12 S13 L113 L114 S14 S15 S16 S17 L115 S18 S19 S20 S21 | L1 L20 L2 L54 | L1 L56 L121 L131 L130 L2 L20 | L1 L19 L2 L58 L127 L126 L125 | L1 L60 L2 L19 | L121 L122 L65 L124 L125 L58 L127 L128 L129 L130 L56 | L56 L130 L131 L121 | L125 L126 L127 L58 | L1 L16 L2 L67 | A1 L17 | L17 A1 | L1 L69 L2 L16 | L1 L15 L2 L71 | L1 L73 L2 L15 | S32 S33 L92 | L92 S33 L135 L136 S34 S35 S36 S37 S38 S39 S40 L137 L138 L139 L140 L141 S41 S42 S43 S31 S32 | L1 L14 L2 L75 | L1 L77 L2 L14 | L1 L13 L2 L79 | L1 L81 L2 L13 | S45 S46 L93 | L93 S46 S47 S48 S49 S50 L142 L143 S51 S52 S53 S54 S55 S44 S45 | L1 L12 L2 L83 | L1 L85 L2 L12 | L1 L11 L2 L87 | L1 L89 L2 L11 | L94 L146 L147 L148 L149 L150 L144 | S63 S64 S65 S66 S67 S68 S69 S70 L151 S71 S72 S73 S74 S75 S76 S77 S78 L152 | S79 S80 S81 S82 S83 S84 S85 S86 L153 S87 S88 S89 S90 S91 S92 S93 S94 L154
body "Solid1"
